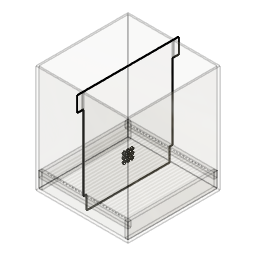
Acrylic Box v6 (Autodesk Fusion 360 design; units mm, degrees)
Autodesk Fusion 360 part; units mm, degrees
sketch "Sketch1" plane through (0, 0, 0) normal (0, 0, 1) x (1, 0, 0)
  line L0 (150, 300) -> (-150, 300)
  line L1 (-150, 300) -> (-150, 0)
  line L2 (-150, 0) -> (150, 0)
  line L3 (150, 0) -> (150, 300)
  line L4 (-145, 295) -> (145, 295)
  line L5 (145, 295) -> (145, 5)
  line L6 (145, 5) -> (-145, 5)
  line L7 (-145, 5) -> (-145, 295)
  dimension "d1" = 300
  dimension "d2" = 300
  dimension "d3" = 5
  dimension "d4" = 5
  dimension "d5" = 5
  dimension "d6" = 5
  constraint horizontal L0
  constraint vertical L1
  constraint horizontal L2
  constraint vertical L3
  constraint midpoint origin L2
  constraint horizontal L4
  constraint vertical L5
  constraint horizontal L6
  constraint vertical L7
  measures "d1" distance of L0.start L0.end
  measures "d2" distance of L0.start L2.end
  measures "d3" distance of L2 L6
  measures "d4" distance of L3 L5
  measures "d5" distance of L1 L7
  measures "d6" distance of L0 L4
extrude "Extrude1" add sketch "Sketch1" along normal blind 350 makes body 1
extrude "Extrude2" add sketch "Sketch1" along normal blind 5 contours L4 L5 L6 L7 bodies 1
sketch "Sketch2" plane through (0, 300, 0) normal (0, 1, 0) x (-1, 0, 0)
  line L0 (-150, 0) -> (150, 0)
  line L1 (150, 0) -> (150, 350)
  line L2 (150, 350) -> (-150, 350)
  line L3 (-150, 350) -> (-150, 0)
  line L4 (-1.5, 350) -> (1.5, 350)
  line L5 (1.5, 350) -> (1.5, 300)
  line L6 (1.5, 300) -> (-1.5, 300)
  line L7 (-1.5, 300) -> (-1.5, 350)
  dimension "d11" = 50
  dimension "d12" = 3
  constraint horizontal L4
  constraint vertical L5
  constraint horizontal L6
  constraint vertical L7
  constraint coincident L2 L4.start
  constraint midpoint L2 L4
  measures "d11" distance of L4.end L5.end
  measures "d12" distance of L5 L7
extrude "Extrude3" cut sketch "Sketch2" against normal blind 300 contours L2 L4 L5 L6 L7 bodies 1
sketch "Sketch3" plane through (0, 295, 0) normal (0, -1, 0) x (1, 0, 0)
  line L0 (1.5, 350) -> (1.5, 300)
  line L1 (1.5, 300) -> (-1.5, 300)
  line L2 (-1.5, 300) -> (-1.5, 350)
  line L3 (-1.5, 350) -> (-145, 350)
  line L4 (-145, 350) -> (-145, 5)
  line L5 (-145, 5) -> (145, 5)
  line L6 (145, 5) -> (145, 350)
  line L7 (145, 350) -> (1.5, 350)
  line L8 (-145, 55) -> (145, 55)
  line L9 (145, 55) -> (145, 35)
  line L10 (145, 35) -> (-145, 35)
  line L11 (-145, 35) -> (-145, 55)
  circle A0 centre (-125, 51) radius 2
  circle A1 centre (-115, 51) radius 2
  circle A2 centre (-105, 51) radius 2
  circle A3 centre (-95, 51) radius 2
  circle A4 centre (-85, 51) radius 2
  circle A5 centre (-75, 51) radius 2
  circle A6 centre (-65, 51) radius 2
  circle A7 centre (-55, 51) radius 2
  circle A8 centre (-45, 51) radius 2
  circle A9 centre (-35, 51) radius 2
  circle A10 centre (-25, 51) radius 2
  circle A11 centre (-15, 51) radius 2
  circle A12 centre (-5, 51) radius 2
  circle A13 centre (5, 51) radius 2
  circle A14 centre (15, 51) radius 2
  circle A15 centre (25, 51) radius 2
  circle A16 centre (35, 51) radius 2
  circle A17 centre (45, 51) radius 2
  circle A18 centre (55, 51) radius 2
  circle A19 centre (65, 51) radius 2
  circle A20 centre (75, 51) radius 2
  circle A21 centre (85, 51) radius 2
  circle A22 centre (95, 51) radius 2
  circle A23 centre (105, 51) radius 2
  circle A24 centre (115, 51) radius 2
  circle A25 centre (125, 51) radius 2
  line L12 (0, 55) -> (0, 0) construction
  line L13 (-145, 5) -> (-135, 5)
  line L14 (-135, 5) -> (-135, 55)
  line L15 (-135, 55) -> (-145, 55)
  line L16 (-145, 55) -> (-145, 5)
  dimension "d15" = 30
  dimension "d16" = 20
  dimension "d17" = 4
  dimension "d22" = 250
  dimension "d23" = 0
  dimension "d24" = 20
  dimension "d25" = 16
  dimension "d31" = 10
  constraint horizontal L8
  constraint vertical L9
  constraint horizontal L10
  constraint vertical L11
  constraint coincident L6 L9.end
  constraint collinear L6 L9
  constraint collinear L4 L11
  constraint midpoint L8 L12.start
  constraint coincident L12.end origin
  constraint horizontal L13
  constraint vertical L14
  constraint horizontal L15
  constraint vertical L16
  constraint coincident L8 L14.end
  constraint coincident L4.end L5.start
  measures "d15" distance of L5 L10
  measures "d16" distance of L8 L10
  measures "d17" diameter of A0
  measures "d24" distance of L11 A0.centre
  measures "d25" distance of L10 A0.centre
  measures "d31" distance of L14 L16
extrude "Extrude4" add sketch "Sketch3" along normal blind 10 separate body contours L6 L8 L9 L10 L14 | L4 L8 L10 L11 L14 L15 L16 | A0 | A1 | A2 | A3 | A4 | A5 | A6 | A7 | A8 | A9 | A10 | A11 | A12 | A13 | A14 | A15 | A16 | A17 | A18 | A19 | A20 | A21 | A22 | A23 | A24 | A25 makes body 2
extrude "Extrude1'" add sketch "Sketch3" along normal blind 290 separate body contours L4 L8 L10 L11 L14 L15 L16 | L4 L5 L10 L13 L14 L16 makes body 3 in component "Grid"
copy_body "CutPasteBodies1" bodies 2 removing the originals makes body 4 in component "Grid"
extrude "Extrude2'" cut sketch "Sketch3" along normal blind 290 contours A0 | A1 | A2 | A3 | A4 | A5 | A6 | A7 | A8 | A9 | A10 | A11 | A12 | A13 | A14 | A15 | A16 | A17 | A18 | A19 | A20 | A21 | A22 | A23 | A24 | A25 bodies 4 in component "Grid"
ref_plane "WorkPlane1" through (0, 150, 175) normal (0, 1, 0) x (-1, 0, 0)
mirror "Mirror1" about plane through (0, 150, 175) normal (0, 1, 0) of bodies 4 makes body 5 in component "Grid"
mirror "Mirror2" about plane through (0, 0, 0) normal (1, 0, 0) of bodies 3 makes body 6 in component "Grid"
extrude "Extrude3'" add sketch "Sketch3" along normal up to surface (290 mm away) contours A0 | A1 | A2 | A3 | A4 | A5 | A6 | A7 | A8 | A9 | A10 | A11 | A12 | A13 | A14 | A15 | A16 | A17 | A18 | A19 | A20 | A21 | A22 | A23 | A24 | A25 bodies 4 5 in component "Grid"
sketch "Sketch1 (2)" plane through (0, 0, 0) normal (1, 0, 0) x (0, 1, 0) in component "Grid"
  line L0 (295, 350) -> (5, 350)
  line L1 (5, 350) -> (5, 55)
  line L2 (5, 55) -> (295, 55)
  line L3 (295, 55) -> (295, 350)
  line L4 (5, 5) -> (5, 350)
  line L5 (295, 5) -> (295, 350)
  line L6 (295, 55) -> (5, 55)
  line L7 (15, 10) -> (285, 10)
  line L8 (285, 10) -> (285, 55)
  line L9 (285, 55) -> (15, 55)
  line L10 (15, 55) -> (15, 10)
  line L11 (1.75, 0) -> (22.5, 0)
  line L12 (15, 35) -> (15, 55)
  line L13 (285, 35) -> (285, 55)
  line L14 (0, 350) -> (300, 350)
  line L15 (5, 350) -> (-15, 350)
  line L16 (-15, 350) -> (-15, 300)
  line L17 (-15, 300) -> (5, 300)
  line L18 (5, 300) -> (5, 350)
  line L19 (5, 300) -> (0, 300)
  line L20 (150, 350) -> (150, -100) construction
  line L21 (295, 300) -> (300, 300)
  line L22 (295, 350) -> (315, 350)
  line L23 (295, 300) -> (295, 350)
  line L24 (315, 350) -> (315, 300)
  line L25 (315, 300) -> (295, 300)
  circle A0 centre (150, 85) radius 5
  circle A1 centre (162.5, 85) radius 5
  circle A2 centre (150, 97.5) radius 5
  circle A3 centre (162.5, 97.5) radius 5
  circle A4 centre (150, 110) radius 5
  circle A5 centre (162.5, 110) radius 5
  circle A6 centre (137.5, 110) radius 5
  circle A7 centre (137.5, 97.5) radius 5
  circle A8 centre (137.5, 85) radius 5
  point P0 (295, 350)
  point P1 (300, 350)
  point P2 (295, 350)
  dimension "d47" = 45
  dimension "d48" = 20
  dimension "d51" = 10
  dimension "d52" = 30
  dimension "d55" = 12.5
  dimension "d56" = 25
  constraint horizontal L0
  constraint vertical L1
  constraint horizontal L2
  constraint vertical L3
  constraint collinear L1 L4
  constraint collinear L3 L5
  constraint collinear L2 L6
  constraint horizontal L7
  constraint vertical L8
  constraint horizontal L9
  constraint vertical L10
  constraint coincident L6 L8.end
  constraint collinear L10 L12
  constraint collinear L8 L13
  constraint collinear L0 L14
  constraint horizontal L15
  constraint vertical L16
  constraint horizontal L17
  constraint vertical L18
  constraint coincident L0.end L1.start
  constraint collinear L17 L19
  constraint midpoint L0 L20.start
  constraint perpendicular L14 L20
  constraint coincident L20 A0.centre
  constraint symmetric L20 A1 A8
  constraint symmetric L20 A3 A7
  constraint symmetric L20 A5 A6
  measures "d47" distance of L7 L9
  measures "d48" distance of L16.end L17.end
  measures "d51" diameter of A0
  measures "d52" distance of L2 A0.centre
extrude "Extrude4'" add sketch "Sketch1 (2)" along normal mid plane 3 separate body contours L0 L1 L2 L3 L4 L5 L6 L9 L14 L18 L23 | L3 L5 L14 L21 L22 L23 L24 L25 | L1 L4 L14 L15 L16 L17 L18 L19 | L2 L6 L7 L8 L9 L10 L12 L13 | A0 | A1 | A2 | A3 | A4 | A5 | A6 | A7 | A8 makes body 7 in component "Grid"
copy_body "Body->Comp1" bodies 7 removing the originals makes body 8 in component "Panel"
extrude "Extrude1''" cut sketch "Sketch1 (2)" along normal mid plane 3 contours A0 | A1 | A2 | A3 | A4 | A5 | A6 | A7 | A8 bodies 8 in component "Panel"
sketch "Dim1" plane through (0, 5, 0) normal (0, -1, 0) x (1, 0, 0) in component "Grid"
  line L0 (-145, 35) -> (145, 35)
  line L1 (145, 35) -> (145, 55)
  line L2 (145, 55) -> (-145, 55)
  line L3 (-145, 55) -> (-145, 35)
  line L4 (145, 5) -> (145, 55)
  line L5 (145, 55) -> (135, 55)
  line L6 (135, 55) -> (135, 5)
  line L7 (135, 5) -> (145, 5)
  line L8 (-145, 55) -> (-145, 5)
  line L9 (-145, 5) -> (-135, 5)
  line L10 (-135, 5) -> (-135, 55)
  line L11 (-135, 55) -> (-145, 55)
  circle A0 centre (-125, 51) radius 2
  circle A1 centre (-115, 51) radius 2
  line L12 (-145, 35) -> (-145, 55)
  point P0 (-125, 51)
  point P1 (-115, 51)
  dimension "d60" = 10
  dimension "d61" = 50
  dimension "d62" = 290
  dimension "d63" = 4
  dimension "d64" = 4
  dimension "d66" = 10
  dimension "d67" = 20
  dimension "d71" = 20
  measures "d60" distance of L8.end L9.end
  measures "d61" distance of L2.end L8.end
  measures "d62" distance of L1.end L2.end
  measures "d63" diameter of A0
  measures "d64" distance of L2 P0
  measures "d66" distance of P0 P1
  measures "d67" distance of P0 L12
  measures "d71" distance of L0 L2
sketch "Dim2" plane through (145, 0, 0) normal (1, 0, 0) x (0, 1, 0) in component "Grid"
  line L0 (295, 5) -> (295, 55)
  line L1 (295, 55) -> (5, 55)
  line L2 (5, 55) -> (5, 5)
  line L3 (5, 5) -> (295, 5)
  line L4 (15, 35) -> (15, 55)
  line L5 (5, 5) -> (5, 55)
  dimension "d68" = 290
  dimension "d69" = 10
  dimension "d70" = 20
  measures "d68" distance of L0.end L1.end
  measures "d69" distance of L4 L5
  measures "d70" distance of L4.start L4.end
sketch "Dim1 (2)" plane through (0, 0, 0) normal (0, -1, 0) x (1, 0, 0)
  line L0 (1.5, 350) -> (1.5, 300)
  line L1 (1.5, 300) -> (-1.5, 300)
  line L2 (-1.5, 300) -> (-1.5, 350)
  line L3 (-1.5, 350) -> (-150, 350)
  line L4 (-150, 350) -> (-150, 0)
  line L5 (-150, 0) -> (150, 0)
  line L6 (150, 0) -> (150, 350)
  line L7 (150, 350) -> (1.5, 350)
  line L8 (-145, 5) -> (-145, 350)
  line L9 (-150, 0) -> (150, 0)
  line L10 (0, 349.9575) -> (0, 250.0425) construction
  dimension "d72" = 3
  dimension "d73" = 50
  dimension "d74" = 350
  dimension "d75" = 5
  dimension "d76" = 300
  dimension "d77" = 150
  constraint perpendicular L7 L10
  constraint midpoint L1 L10
  measures "d72" distance of L0 L2
  measures "d73" distance of L1.end L2.end
  measures "d74" distance of L3.end L4.end
  measures "d75" distance of L4 L8
  measures "d76" distance of L4.end L5.end
  measures "d77" distance of L4 L10
sketch "Sketch1 (3)" plane through (1.5, 0, 0) normal (1, 0, 0) x (0, 1, 0) in component "Panel"
  circle A0 centre (150, 97.5) radius 5
  circle A1 centre (162.5, 110) radius 5
  circle A2 centre (150, 110) radius 5
  circle A3 centre (162.5, 85) radius 5
  circle A4 centre (137.5, 85) radius 5
  circle A5 centre (137.5, 110) radius 5
  circle A6 centre (162.5, 97.5) radius 5
  circle A7 centre (150, 85) radius 5
  circle A8 centre (137.5, 97.5) radius 5
  line L0 (315, 350) -> (-15, 350)
  line L1 (-15, 350) -> (-15, 300)
  line L2 (-15, 300) -> (5, 300)
  line L3 (5, 300) -> (5, 55)
  line L4 (5, 55) -> (15, 55)
  line L5 (15, 55) -> (15, 10)
  line L6 (15, 10) -> (285, 10)
  line L7 (285, 10) -> (285, 55)
  line L8 (285, 55) -> (295, 55)
  line L9 (295, 55) -> (295, 300)
  line L10 (295, 300) -> (315, 300)
  line L11 (315, 300) -> (315, 350)
  line L12 (15, 10) -> (285, 10)
  line L13 (15, 55) -> (15, 10)
  line L14 (5, 350) -> (5, 55)
  line L15 (315, 350) -> (315, 300)
  line L16 (-15, 350) -> (-15, 300)
  line L17 (5, 300) -> (5, 350)
  line L18 (5, 55) -> (295, 55)
  line L19 (285, 55) -> (15, 55)
  point P0 (137.5, 85)
  point P1 (150, 85)
  dimension "d78" = 50
  dimension "d79" = 245
  dimension "d80" = 45
  dimension "d81" = 12.5
  dimension "d82" = 10
  dimension "d83" = 12.5
  dimension "d84" = 270
  dimension "d85" = 10
  dimension "d86" = 330
  dimension "d87" = 20
  dimension "d89" = 30
  measures "d78" distance of L0.end L1.end
  measures "d79" distance of L2 L4
  measures "d80" distance of L4.end L5.end
  measures "d81" distance of A5.centre A8.centre
  measures "d82" diameter of A5
  measures "d83" distance of A2.centre A5.centre
  measures "d84" distance of L5.end L6.end
  measures "d85" distance of L13 L14
  measures "d86" distance of L15 L16
  measures "d87" distance of L16 L17
  measures "d89" distance of P1 L19
component "Grid" placed x (1, 0, 0) y (0, 1, 0) z (0, 0, 1) at (0, 0, 0)
component "Panel" placed x (1, 0, 0) y (0, 1, 0) z (0, 0, 1) at (0, 0, 0)
